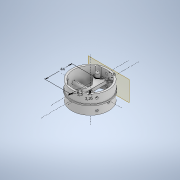
# Autodesk Inventor part: Verbindungsring_bottom
Saved by Autodesk Inventor 2020 (Build 240168000, 168)
## iProperties
Created: 2022-02-05
Part Number: Verbindungsring_bottom
Material: Generisch
Document SubType Name: Modeling
Designer: sp
Density: 1 g/cm^3
Appearance: Vorgabe
Author: sp
## iProperties of the stored document _3D-Druck.ipt
Created: 2022-05-01
Part Number: _3D-Druck
Material: Generisch
Document SubType Name: Modeling
Designer: sp
Density: 1 g/cm^3
Appearance: Vorgabe
Author: sp
Autodesk Inventor part; units mm, degrees
ref_plane "YZ Plane" through (0, 0, 0) normal (1, 0, 0) x (0, 1, 0)
ref_plane "XZ Plane" through (0, 0, 0) normal (0, 1, 0) x (-1, 0, 0)
sketch "Skizze5" plane through (0, 0, 0) normal (0, 1, 0) x (-1, 0, 0)
  circle A0 centre (0, 0) radius 27
  circle A1 centre (0, 0) radius 31
  dimension "d23" = 62
  dimension "d24" = 54
  constraints: 2 centre point, 2 coincident
  measures "d23" diameter of A1
  measures "d24" diameter of A0
extrude "Extrusion4" add sketch "Skizze5" along normal mid plane 2
sketch "Skizze6" plane through (0, 0, 0) normal (0, 1, 0) x (-1, 0, 0)
  circle A0 centre (0, 0) radius 27
  circle A1 centre (0, 0) radius 30
  dimension "d27" = 54
  dimension "d28" = 60
  constraints: 2 centre point, 2 coincident
  measures "d27" diameter of A0
  measures "d28" diameter of A1
extrude "Extrusion5" add sketch "Skizze6" along normal mid plane 30
ref_plane "Arbeitsebene5" through (0, 0, -30) normal (0, 0, 1) x (1, 0, 0)
sketch "Skizze7" plane through (0, 0, -30) normal (0, 0, 1) x (1, 0, 0)
  circle A0 centre (0, -9) radius 1.75
  circle A1 centre (0, 9) radius 1.75
  line L0 (-34.501484, 0) -> (40.45081, 0) construction
  point P0 (0, 0)
  dimension "d32" = 3.5
  dimension "d33" = 3.5
  dimension "d34" = 18
  constraints: 2 centre point, 2 end point, 1 horizontal, 1 point on line, 1 symmetric about line
  measures "d32" diameter of A0
  measures "d33" diameter of A1
  measures "d34" distance of A1.centre A0.centre
extrude "Extrusion6" cut sketch "Skizze7" along normal blind 5
pattern_circular "Runde Anordnung2" count 3 over 360 about axis through (0, -10, 0) along (0, 1, 0) of "Extrusion6"
sketch "Skizze14" plane through (0, 0, 0) normal (0, 1, 0) x (-1, 0, 0)
  line L0 (2.5, -29.75) -> (-2.5, -29.75)
  line L1 (-2.5, -29.75) -> (-2.5, 29.75)
  line L2 (-2.5, 29.75) -> (2.5, 29.75)
  line L3 (2.5, 29.75) -> (2.5, -29.75)
  line L4 (0, -26.188119) -> (0, 26.188119) construction
  line L5 (10.744199, 0) -> (-15.592863, 0) construction
  point P0 (0, 0)
  point P1 (0, 0)
  dimension "d77" = 5
  dimension "d78" = 59.5
  constraints: 12 end point, 2 horizontal, 2 midpoint, 2 parallel, 2 point on line, 1 perpendicular, 1 vertical, 2 other
  measures "d77" distance between parallel lines of L1 L3
  measures "d78" distance between parallel lines of L0 L2
extrude "Extrusion13" add sketch "Skizze14" along normal mid plane 5
sketch "Skizze15" plane through (0, 0, 0) normal (0, 1, 0) x (-1, 0, 0)
  line L0 (0, 80.260451) -> (0, -80.55427) construction
  line L1 (48.234625, 0) -> (-52.543911, 0) construction
  circle A0 centre (10, 22) radius 4.25
  circle A1 centre (10, -22) radius 4.25
  line L2 (10, 55.579994) -> (10, -73.992403) construction
  circle A2 centre (10, 22) radius 2.75
  circle A3 centre (10, -22) radius 2.75
  point P0 (0, 0)
  dimension "d81" = 8.5
  dimension "d82" = 8.5
  dimension "d83" = 10
  dimension "d84" = 44
  dimension "d85" = 5.5
  dimension "d86" = 5.5
  constraints: 6 end point, 4 centre point, 3 point on line, 2 coincident, 2 vertical, 1 horizontal, 1 symmetric about line
  measures "d81" diameter of A0
  measures "d82" diameter of A1
  measures "d83" distance between parallel lines of L0 L2
  measures "d84" distance of A0.centre A1.centre
  measures "d85" diameter of A2
  measures "d86" diameter of A3
extrude "Extrusion14" add sketch "Skizze15" along normal blind 10 contours A2 | A3
sketch "Skizze17" plane through (0, 0, 0) normal (0, 1, 0) x (-1, 0, 0)
  circle A0 centre (10, 22) radius 2.75
  circle A1 centre (10, 22) radius 5
  circle A2 centre (10, -22) radius 2.75
  circle A3 centre (10, -22) radius 5
  line L0 (13.754093, -18.697458) -> (2.5, -5.851948)
  line L1 (5.9941, -24.992117) -> (2.5, -20.017832)
  line L2 (2.5, -20.017832) -> (2.5, -5.851948)
  line L3 (2.5, 26.88401) -> (2.5, -26.88401)
  line L4 (5.476936, 24.131171) -> (2.5, 17.836262)
  line L5 (14.188209, 19.268901) -> (2.5, 5.028767)
  line L6 (2.5, 5.028767) -> (2.5, 17.836262)
  point P0 (0, 0)
  point P1 (10.217343, 24.992117)
  point P2 (12.111424, 24.131171)
  point P3 (12.111424, -24.131171)
  point P4 (10.217343, -24.992117)
  point P5 (5.826426, -24.753413)
  point P6 (13.495211, 18.424598)
  dimension "d89" = 10
  dimension "d90" = 10
  constraints: 12 end point, 4 point on circle, 2 centre point, 2 coincident, 2 collinear, 2 point on line, 2 other
  measures "d89" diameter of A1
  measures "d90" diameter of A3
sketch "Skizze17 outline for Extrusion15" plane through (0, 0, 0) normal (0, 1, 0) x (-1, 0, 0)
  line L0 (2.5, -5.851948) -> (2.5, -20.017832)
  line L1 (13.754093, -18.697458) -> (2.5, -5.851948)
  arc A0 (5.826426, -24.753413) -> (13.754093, -18.697458) centre (10, -22) ccw
  line L2 (2.5, -20.017832) -> (5.826426, -24.753413)
  arc A1 (13.495211, 18.424598) -> (5.476936, 24.131171) centre (10, 22) ccw
  line L3 (2.5, 5.028767) -> (13.495211, 18.424598)
  line L4 (2.5, 17.836262) -> (2.5, 5.028767)
  line L5 (5.476936, 24.131171) -> (2.5, 17.836262)
extrude "Extrusion15" add sketch "Skizze17 outline for Extrusion15" along normal mid plane 5
extrude "Extrusion16" cut sketch "Skizze15" along normal blind 15
fillet "Rundung8" radius 1 2 edges at (-2.5, 0, 17.8363) (-2.5, 0, -20.0178)
fillet "Rundung9" radius 1 16 edges at (-7.0764, 1.75, -26.0562) (-7.0764, -1.75, -26.0562) (-14.9784, -1.75, -22.4644) (-7.0764, 0.5, -26.0562) (-7.0764, -0.5, -26.0562) (-14.9784, 1.75, -22.4644) (-14.9784, 0.5, -22.4644) (-14.9784, -0.5, -22.4644) (-7.0764, 1.75, 26.0562) (-7.0764, 0.5, 26.0562) (-7.0764, -0.5, 26.0562) (-7.0764, -1.75, 26.0562) (-14.9784, -1.75, 22.4644) (-14.9784, -0.5, 22.4644) (-14.9784, 0.5, 22.4644) (-14.9784, 1.75, 22.4644)
sketch "Skizze18" plane through (0, 10, 0) normal (0, 1, 0) x (1, 0, 0)
  circle A0 centre (-10, -22) radius 2.75 projected
  circle A1 centre (-10, -22) radius 3
  circle A2 centre (-10, 22) radius 2.75 projected
  circle A3 centre (-10, 22) radius 3
  point P0 (0, 0)
  constraints: 2 centre point, 2 coincident
extrude "Extrusion17" cut sketch "Skizze18" along normal blind 15 contours A0 | A2
fillet "Rundung10" radius 2 2 edges at (-7.25, 10, 22) (-7.25, 10, -22)
sketch "Skizze19" plane through (0, 0, 0) normal (1, 0, 0) x (0, 1, 0)
  line L0 (49.382499, 0) -> (-50.664372, 0) construction
  line L1 (-3, -35.734569) -> (-3, 36.806964) construction
  circle A0 centre (-3, 0) radius 1.6
  circle A1 centre (-3, 0) radius 3
  point P0 (0, 0)
  dimension "d100" = 3
  dimension "d101" = 3.2
  dimension "d102" = 6
  constraints: 4 end point, 3 point on line, 2 centre point, 1 coincident, 1 horizontal, 1 vertical
  measures "d100" distance from line of point (0, 0) L1
  measures "d101" diameter of A0
  measures "d102" diameter of A1
extrude "Extrusion18" add sketch "Skizze19" along normal mid plane 59.6
extrude "Extrusion19" cut sketch "Skizze19" along normal mid plane 65 contours A0
